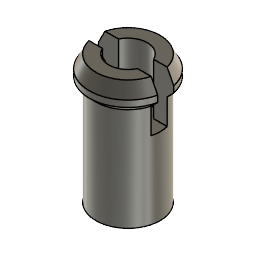
Peg Connection_v1 (Autodesk Fusion 360 design; units mm, degrees)
part number: 2026-01-19-14-38-02-559
Autodesk Fusion 360 part; units mm, degrees
note: some values were not read from the file. Set by a fixed rule: which sketch regions a step uses.
sketch "Sketch2" plane through (0, 0, 0) normal (0, 1, 0) x (1, 0, 0)
  line L0 (0, 0) -> (12.7, 0)
  line L1 (12.7, 0) -> (12.7, -15.24)
  line L2 (15.24, -15.24) -> (15.24, -25.4)
  line L3 (12.7, -25.4) -> (7.62, -25.4)
  line L4 (7.62, -25.4) -> (7.62, -5.08)
  line L5 (7.62, -5.08) -> (0, -5.08)
  line L6 (0, -1.75) -> (0, -22.5)
  line L7 (0, -5.08) -> (0, 0)
  line L8 (12.7, -25.4) -> (15.24, -25.4)
  line L9 (12.7, -15.24) -> (15.24, -15.24)
  dimension "d9" = 12.7
  dimension "d11" = 5.08
  dimension "d12" = 5.08
  dimension "d14" = 5.08
  dimension "d15" = 25.4
  dimension "d16" = 10.16
  dimension "d22" = 7.62
  constraint coincident L0.start L7.end
  constraint horizontal L0
  constraint perpendicular L0 L1
  constraint perpendicular L0 L2
  constraint perpendicular L2 L3
  constraint perpendicular L3 L4
  constraint perpendicular L4 L5
  constraint coincident L5.end L6
  constraint perpendicular L2 L8
  constraint perpendicular L2 L9
  measures "d9" distance of L1 L6
  measures "d11" distance of L0 L5
  measures "d12" distance of L1 L4
  measures "d14" distance of L3.start L3.end
  measures "d15" distance of L0 L3
  measures "d16" distance of L2.start L2.end
  measures "d22" distance of L2 L4
revolve "Revolve1" add sketch "Sketch2" angle 360 about axis through (0, 0, 1.75) along (0, 0, 1)
sketch "Sketch3" plane through (0, 0, 25.4) normal (0, 0, 1) x (-1, 0, 0)
  circle A0 centre (0, 0) radius 7.62
  line L0 (19.05, -3.175) -> (-19.05, -3.175)
  line L1 (-19.05, -3.175) -> (-19.05, 3.175)
  line L2 (-19.05, 3.175) -> (19.05, 3.175)
  line L3 (19.05, 3.175) -> (19.05, -3.175)
  line L4 (-1.75, 0) -> (-22.5, 0)
  line L5 (0, -1.75) -> (0, -22.5)
  circle A1 centre (0, 0) radius 15.24
  dimension "d18" = 6.35
  dimension "d19" = 38.1
  constraint horizontal L0
  constraint vertical L1
  constraint horizontal L2
  constraint vertical L3
  constraint symmetric L0 L2 L4
  constraint symmetric L1 L3 L5
  measures "d18" distance of L0 L2
  measures "d19" distance of L1 L3
extrude "Extrude2" cut sketch "Sketch3" against normal blind 20.32 contours A0 L0 L2 | A0 L0 L2 A1 | A0 L2 L4 A1 | L0 L2 L3 A1 | A0 L0 L4 A1 | L1 L2 L4 A1 | L0 L1 L4 A1
chamfer "Chamfer1" distance 2.54 distance2 5.08 2 edges at (0, -15.24, 25.4) (0, 15.24, 25.4) measured on face at (0, -12.6739, 25.4) measured on face at (0, 12.6739, 25.4)
chamfer "Chamfer1" distance 2.54 angle 45 2 edges at (0, -15.24, 15.24) (0, 15.24, 15.24)
extrude "Extrude3" add 1 faces at (4.7561, -2.479, 0) along direction (0, 0, -1) blind 25.4
